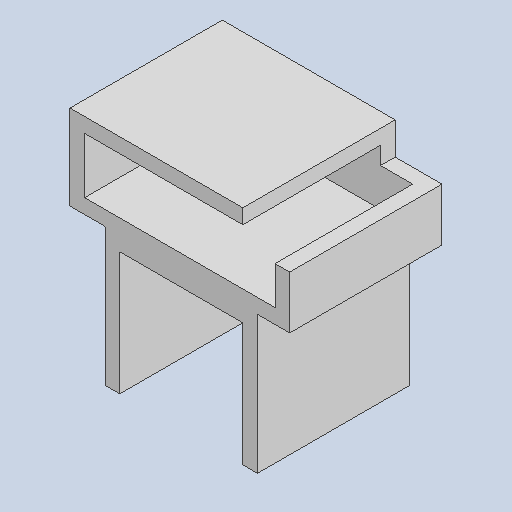
# Autodesk Inventor part: new_camera_case_front
Saved by Autodesk Inventor 2025.2 (Build 292293000, 293)
## iProperties
Created: 2025-05-20
Part Number: new_camera_case_front
Material: 일반
Document SubType Name: Modeling
Designer: jbhma
Density: 1 g/cm^3
Appearance: 기본값
Author: jbhma
Autodesk Inventor part; units mm, degrees
ref_plane "YZ Plane" through (0, 0, 0) normal (1, 0, 0) x (0, 1, 0)
ref_plane "XZ Plane" through (0, 0, 0) normal (0, 1, 0) x (-1, 0, 0)
ref_plane "XY Plane" through (0, 0, 0) normal (0, 0, 1) x (1, 0, 0)
sketch "스케치1" plane through (0, 0, 0) normal (0, 1, 0) x (-1, 0, 0)
  line L0 (24.089, 25.4241) -> (-27.911, 25.4241)
  line L1 (-27.911, 25.4241) -> (-27.911, -26.5759)
  line L2 (-27.911, -26.5759) -> (24.089, -26.5759)
  line L3 (24.089, -26.5759) -> (24.089, 25.4241)
  point P0 (0, 0)
  dimension "d0" = 52
  dimension "d1" = 52
  constraints: 8 end point, 2 parallel, 1 coincident, 1 horizontal, 1 perpendicular
  measures "d0" distance of L2.end L1.end
  measures "d1" distance of L1.end L0.end
extrude "돌출2" add sketch "스케치1" along normal blind 5
sketch "스케치2" plane through (0, 0, 0) normal (0, -1, 0) x (1, 0, 0)
  line L0 (27.911, 25.4241) -> (27.911, -26.5759) projected
  line L1 (-24.089, 25.4241) -> (27.911, 25.4241) projected
  line L2 (-24.089, -26.5759) -> (-24.089, 25.4241) projected
  line L3 (27.911, -26.5759) -> (-24.089, -26.5759) projected
  line L4 (-24.089, 25.4241) -> (-19.089, 25.4241)
  line L5 (-19.089, 25.4241) -> (-19.089, -26.5759)
  line L6 (-19.089, -26.5759) -> (-24.089, -26.5759)
  line L7 (-24.089, -26.5759) -> (-24.089, 25.4241)
  line L8 (27.911, 25.4241) -> (22.911, 25.4241)
  line L9 (22.911, 25.4241) -> (22.911, -26.5759)
  line L10 (22.911, -26.5759) -> (27.911, -26.5759)
  line L11 (27.911, -26.5759) -> (27.911, 25.4241)
  point P0 (0, 0)
  dimension "d8" = 5
  dimension "d9" = 5
  constraints: 16 end point, 4 parallel, 2 horizontal, 2 perpendicular, 2 point on line
  measures "d8" distance of L5.end L6.end
  measures "d9" distance of L10.end L9.end
extrude "돌출3" add sketch "스케치2" along normal blind 42 contours L0 L3 L9 L1 | L5 L3 L2 L1
sketch "스케치3" plane through (0, 5, 0) normal (0, 1, 0) x (1, 0, 0)
  point P0 (0, 0)
sketch "스케치4" plane through (0, 5, 0) normal (0, 1, 0) x (1, 0, 0)
  line L0 (27.911, -25.4241) -> (27.911, 26.5759) projected
  line L1 (27.911, 26.5759) -> (-24.089, 26.5759) projected
  line L2 (-24.089, 26.5759) -> (-24.089, -25.4241) projected
  line L3 (-24.089, -25.4241) -> (27.911, -25.4241) projected
  line L4 (27.911, 26.5759) -> (38.911, 26.5759)
  line L5 (38.911, 26.5759) -> (38.911, -25.4241)
  line L6 (38.911, -25.4241) -> (27.911, -25.4241)
  line L7 (27.911, -25.4241) -> (27.911, 26.5759)
  line L8 (-24.089, 26.5759) -> (-36.089, 26.5759)
  line L9 (-36.089, 26.5759) -> (-36.089, -25.4241)
  line L10 (-36.089, -25.4241) -> (-24.089, -25.4241)
  line L11 (-24.089, -25.4241) -> (-24.089, 26.5759)
  line L12 (-24.089, 26.5759) -> (27.911, 26.5759)
  line L13 (27.911, 26.5759) -> (27.911, -25.4241)
  line L14 (27.911, -25.4241) -> (-24.089, -25.4241)
  line L15 (-24.089, -25.4241) -> (-24.089, 26.5759)
  point P0 (0, 0)
  point P1 (-24.089, -25.4241)
  dimension "d12" = 11
  dimension "d13" = 12
  constraints: 24 end point, 6 parallel, 3 horizontal, 3 perpendicular
  measures "d12" distance of L5.end L6.end
  measures "d13" distance of L10.end L9.end
extrude "돌출4" add sketch "스케치4" along normal blind 5
sketch "스케치5" plane through (0, 10, 0) normal (0, 1, 0) x (1, 0, 0)
  line L0 (-36.089, -25.4241) -> (38.911, -25.4241) projected
  line L1 (38.911, -25.4241) -> (38.911, 26.5759) projected
  line L2 (38.911, 26.5759) -> (-36.089, 26.5759) projected
  line L3 (-36.089, 26.5759) -> (-36.089, -25.4241) projected
  line L4 (-36.089, 26.5759) -> (-31.089, 26.5759)
  line L5 (-31.089, 21.5759) -> (-31.089, -25.4241)
  line L6 (-31.089, -25.4241) -> (-36.089, -25.4241)
  line L7 (-36.089, -25.4241) -> (-36.089, 26.5759)
  line L8 (38.911, 26.5759) -> (33.911, 26.5759)
  line L9 (33.911, 21.5759) -> (33.911, -25.4241)
  line L10 (33.911, -25.4241) -> (38.911, -25.4241)
  line L11 (38.911, -25.4241) -> (38.911, 26.5759)
  line L12 (-36.089, 26.5759) -> (38.911, 26.5759)
  line L13 (38.911, 26.5759) -> (38.911, 21.5759)
  line L14 (33.911, 21.5759) -> (-31.089, 21.5759)
  line L15 (-36.089, 21.5759) -> (-36.089, 26.5759)
  point P0 (0, 0)
  dimension "d16" = 5
  dimension "d17" = 5
  dimension "d18" = 5
  constraints: 24 end point, 6 parallel, 3 horizontal, 3 perpendicular, 3 point on line
  measures "d16" distance of L5.end L6.end
  measures "d17" distance of L10.end L9.end
  measures "d18" distance of L12.end L13.end
extrude "돌출5" add sketch "스케치5" along normal blind 13 contours L3 L2 L1 L0 L9 L14 L5
sketch "스케치6" plane through (0, 23, 0) normal (0, 1, 0) x (1, 0, 0)
  line L0 (33.911, 21.5759) -> (33.911, -25.4241) projected
  line L1 (33.911, -25.4241) -> (38.911, -25.4241) projected
  line L2 (38.911, -25.4241) -> (38.911, 26.5759) projected
  line L3 (38.911, 26.5759) -> (-36.089, 26.5759) projected
  line L4 (-36.089, 26.5759) -> (-36.089, -25.4241) projected
  line L5 (-36.089, -25.4241) -> (-31.089, -25.4241) projected
  line L6 (-31.089, -25.4241) -> (-31.089, 21.5759) projected
  line L7 (-31.089, 21.5759) -> (33.911, 21.5759) projected
  line L8 (38.911, 26.5759) -> (22.911, 26.5759)
  line L9 (22.911, 26.5759) -> (22.911, 21.5759)
  line L10 (22.911, 21.5759) -> (38.911, 21.5759)
  line L11 (38.911, 21.5759) -> (38.911, 26.5759)
  point P0 (0, 0)
  dimension "d21" = 16
  constraints: 8 end point, 2 parallel, 1 horizontal, 1 perpendicular, 1 point on line
  measures "d21" distance of L10.end L9.end
extrude "돌출6" add sketch "스케치6" along normal blind 11 contours L7 L6 L5 L4 L3 L9
sketch "스케치7" plane through (-31.089, 10, 25.4241) normal (1, 0, 0) x (0, 0, -1)
  line L0 (47, 0) -> (0, 0) projected
  line L1 (47, 0) -> (47, 24) projected
  line L2 (0, 24) -> (47, 24) projected
  line L3 (0, 0) -> (0, 24) projected
  line L4 (0, 24) -> (47, 24)
  line L5 (47, 24) -> (47, 19)
  line L6 (47, 19) -> (0, 19)
  line L7 (0, 19) -> (0, 24)
  point P0 (25.4241, -10)
  point P1 (0, 19)
  constraints: 8 end point, 2 parallel, 1 horizontal, 1 perpendicular, 1 point on line
extrude "돌출7" add sketch "스케치7" along normal blind 54 contours L6 L3 L2 L1
